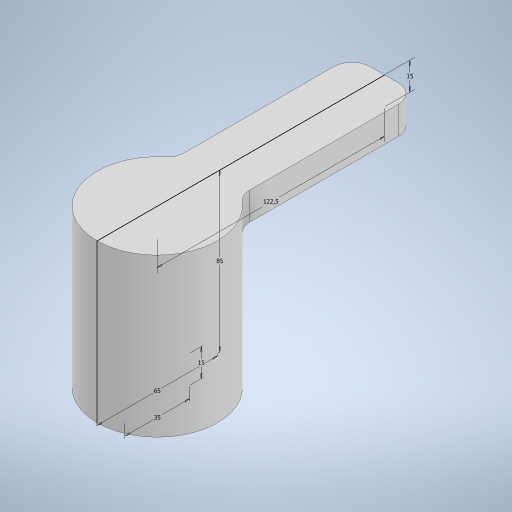
# Autodesk Inventor part: Wkp 01.03.2
Saved by Autodesk Inventor 2023 (Build 270158000, 158)
## iProperties
Created: 2023-03-01
Part Number: Wkp 01.03.2
Material: Generic
Document SubType Name: Modeling
Designer: accam
Density: 1 g/cm^3
Appearance: Default
Author: accam
Autodesk Inventor part; units mm, degrees
ref_plane "YZ Plane" through (0, 0, 0) normal (1, 0, 0) x (0, 1, 0)
ref_plane "XZ Plane" through (0, 0, 0) normal (0, 1, 0) x (-1, 0, 0)
ref_plane "XY Plane" through (0, 0, 0) normal (0, 0, 1) x (1, 0, 0)
sketch "Sketch1" plane through (0, 0, 0) normal (1, 0, 0) x (0, 1, 0)
  line L0 (42.5, 32.5) -> (-42.5, 32.5)
  line L1 (-42.5, 32.5) -> (-42.5, -32.5)
  line L2 (-42.5, -32.5) -> (42.5, -32.5)
  line L3 (42.5, -32.5) -> (42.5, 32.5)
  line L4 (42.5, 32.5) -> (-42.5, -32.5) construction
  line L5 (-42.5, 32.5) -> (42.5, -32.5) construction
  line L6 (-35, 17.5) -> (-50, 17.5)
  line L7 (-50, 17.5) -> (-50, -17.5)
  line L8 (-50, -17.5) -> (-35, -17.5)
  line L9 (-35, -17.5) -> (-35, 17.5)
  line L10 (-35, 17.5) -> (-50, -17.5) construction
  line L11 (-50, 17.5) -> (-35, -17.5) construction
  line L12 (42.5, 0) -> (-50, 0)
  line L13 (42.5, 0) -> (27.5, 0)
  line L14 (27.5, 0) -> (27.5, -122.5)
  line L15 (27.5, -122.5) -> (42.5, -122.5)
  line L16 (42.5, -122.5) -> (42.5, 0)
  point P0 (0, 0)
  point P1 (-42.5, 0)
  point P2 (-42.5, -17.5)
  dimension "d0" = 85
  dimension "d1" = 65
  dimension "d2" = 15
  dimension "d3" = 35
  dimension "d5" = 15
  dimension "d6" = 122.5
  constraints: 34 end point, 7 midpoint, 6 parallel, 3 horizontal, 3 perpendicular
  measures "d0" distance of L2.end L1.end
  measures "d1" distance of L1.end L0.end
  measures "d2" distance of L8.end L7.end
  measures "d3" distance of L7.end L6.end
  measures "d5" distance of L15.end L14.end
  measures "d6" distance of L14.end L13.end
revolve "Revolution1" add sketch "Sketch1" angle 360 mid plane about axis through (0, 42.5, 0) along (0, -1, 0) contours L3 L2 L14 L12 | L14 L2 L1 L8 L9 L12 | L12 L9 L8 L1 | L1 L8 L7 L12
extrude "Extrusion1" add sketch "Sketch1" along normal mid plane 35 contours L3 L2 L14 L12 | L16 L15 L14 L2
fillet "Fillet1" radius 10 2 edges at (17.5, 35, -27.3861) (-17.5, 35, -27.3861)
fillet "Fillet2" radius 10 2 edges at (17.5, 35, -122.5) (-17.5, 35, -122.5)
body "Solid1"
